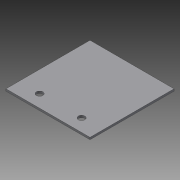
# Autodesk Inventor part: gard
Saved by Autodesk Inventor 2015 (Build 190159000, 159)
## iProperties
Created: 2015-12-11
Part Number: gard
Material: 一般
Document SubType Name: Modeling
Designer: kenta
Density: 1 g/cm^3
Appearance: 既定
Author: kenta
Autodesk Inventor part; units mm, degrees
ref_plane "YZ Plane" through (0, 0, 0) normal (1, 0, 0) x (0, 1, 0)
ref_plane "XZ Plane" through (0, 0, 0) normal (0, 1, 0) x (-1, 0, 0)
ref_plane "XY Plane" through (0, 0, 0) normal (0, 0, 1) x (1, 0, 0)
sketch "スケッチ1" plane through (0, 0, 0) normal (0, 0, 1) x (1, 0, 0)
  line L0 (-20, 20) -> (20, 20)
  line L1 (20, 20) -> (20, -20)
  line L2 (20, -20) -> (-20, -20)
  line L3 (-20, -20) -> (-20, 20)
  line L4 (-20, 20) -> (20, -20) construction
  line L5 (20, 20) -> (-20, -20) construction
  point P0 (0, 0)
  dimension "d0" = 40
  dimension "d1" = 40
  constraints: 12 end point, 2 midpoint, 2 parallel, 1 horizontal, 1 perpendicular
  measures "d0" distance of L1.end L2.end
  measures "d1" distance of L0.end L1.end
extrude "押し出し1" add sketch "スケッチ1" along normal blind 1
sketch "スケッチ2" plane through (0, 0, 1) normal (0, 0, 1) x (1, 0, 0)
  line L0 (-20, 20) -> (-20, -20) projected
  line L1 (20, -20) -> (20, 20) projected
  line L2 (-20, -20) -> (20, -20) projected
  circle A0 centre (-10, -14) radius 1.55
  circle A1 centre (10, -14) radius 1.55
  point P0 (0, 0)
  dimension "d4" = 10
  dimension "d5" = 10
  dimension "d6" = 6
  dimension "d7" = 6
  dimension "d8" = 3.1
  dimension "d9" = 3.1
  constraints: 2 centre point, 2 coincident
  measures "d4" distance from line of point (-10, -14) L0
  measures "d5" distance from line of point (10, -14) L1
  measures "d6" distance from line of point (10, -14) L2
  measures "d7" distance from line of point (-10, -14) L2
  measures "d8" diameter of A0
  measures "d9" diameter of A1
extrude "押し出し2" cut sketch "スケッチ2" against normal blind 1
